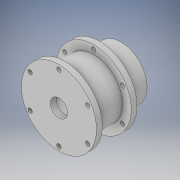
# Autodesk Inventor part: PreCombChamber4_4
Saved by Autodesk Inventor 2017 (Build 210142000, 142)
## iProperties
Created: 2018-04-05
Part Number: PreCombChamber4_4
Material: Generic
Document SubType Name: Modeling
Designer: Johnny
Density: 1 g/cm^3
Appearance: Default
Author: Johnny
Autodesk Inventor part; units mm, degrees
ref_plane "YZ Plane" through (0, 0, 0) normal (1, 0, 0) x (0, 1, 0)
ref_plane "XZ Plane" through (0, 0, 0) normal (0, 1, 0) x (-1, 0, 0)
ref_plane "XY Plane" through (0, 0, 0) normal (0, 0, 1) x (1, 0, 0)
sketch "Sketch1" plane through (0, 0, 0) normal (0, 0, 1) x (1, 0, 0)
  circle A0 centre (0, 0) radius 41.148
  dimension "d0" = 82.296
  constraints: 1 centre point, 1 coincident
  measures "d0" diameter of A0
extrude "Extrusion1" add sketch "Sketch1" against normal blind 68.072
sketch "Sketch2" plane through (0, 0, 0) normal (0, 0, 1) x (1, 0, 0)
  circle A0 centre (0, 0) radius 9.525
  dimension "d3" = 19.05
  constraints: 1 centre point, 1 coincident
  measures "d3" diameter of A0
extrude "Extrusion2" cut sketch "Sketch2" against normal blind 68.072
sketch "Sketch3" plane through (0, 0, -68.072) normal (0, 0, -1) x (-1, 0, 0)
  circle A0 centre (0, 0) radius 21.844
  dimension "d6" = 43.688
  constraints: 1 centre point, 1 coincident
  measures "d6" diameter of A0
extrude "Extrusion3" cut sketch "Sketch3" against normal blind 23.622
sketch "Sketch4" plane through (0, 0, 0) normal (0, 0, 1) x (1, 0, 0)
  circle A0 centre (0, 0) radius 9.525
  constraints: 1 centre point, 1 coincident
extrude "Extrusion4" add sketch "Sketch4" against normal blind 6.35
loft "Loft1" cut section 1 edges at (-9.525, 0, -6.35) section 2 edges at (21.844, 0, -44.45)
sketch "Sketch5" plane through (0, 0, 0) normal (0, 0, 1) x (1, 0, 0)
  point P0 (0, 0)
hole "Hole1" at (0, 0, 0) direction (0, 0, -1) diameter 19.05 depth 50.419 tip angle 118
sketch "Sketch6" plane through (0, 0, 0) normal (0, 0, 1) x (1, 0, 0)
  circle A0 centre (0, 0) radius 41.148
  circle A1 centre (0, 0) radius 31.75
  dimension "d22" = 63.5
  constraints: 2 centre point, 2 coincident
  measures "d22" diameter of A1
sketch "Sketch7" plane through (0, 0, -68.072) normal (0, 0, -1) x (-1, 0, 0)
  circle A0 centre (0, 0) radius 41.148
  circle A1 centre (0, 0) radius 9.525 projected
  circle A2 centre (0, 0) radius 28.575
  dimension "d23" = 57.15
  constraints: 2 centre point, 2 coincident
  measures "d23" diameter of A2
extrude "Extrusion5" cut sketch "Sketch7" against normal blind 23.622 contours A0
extrude "Extrusion6" cut sketch "Sketch6" against normal blind 38.1
sketch "Sketch8" plane through (0, 0, 0) normal (0, 0, 1) x (1, 0, 0)
  circle A0 centre (0, 0) radius 31.75
  circle A1 centre (0, 0) radius 41.148
  constraints: 2 centre point, 2 coincident
extrude "Extrusion7" add sketch "Sketch8" against normal blind 6.35
sketch "Sketch9" plane through (0, 0, 0) normal (0, 0, 1) x (1, 0, 0)
  circle A0 centre (0, 36.449) radius 2.3812
  circle A1 centre (31.5658, 18.2245) radius 2.3812
  circle A2 centre (31.5658, -18.2245) radius 2.3812
  circle A3 centre (0, -36.449) radius 2.3812
  circle A4 centre (-31.5658, -18.2245) radius 2.3812
  circle A5 centre (-31.5658, 18.2245) radius 2.3812
  point P0 (0, 0)
  dimension "d30" = 4.7625
  dimension "d33" = 360
  constraints: 6 centre point, 13 other
  measures "d30" diameter of A0
extrude "Extrusion8" cut sketch "Sketch9" against normal blind 127
body "Solid1"
